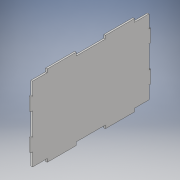
# Autodesk Inventor part: rev1 large wall
Saved by Autodesk Inventor 2017 (Build 210142000, 142)
## iProperties
Created: 2019-05-03
Part Number: rev1 large wall
Material: Generic
Document SubType Name: Modeling
Designer: Roman
Density: 1 g/cm^3
Appearance: Default
Author: Roman
Autodesk Inventor part; units mm, degrees
ref_plane "YZ Plane" through (0, 0, 0) normal (1, 0, 0) x (0, 1, 0)
sketch "Sketch1" plane through (0, 0, 0) normal (1, 0, 0) x (0, 1, 0)
  line L0 (0, 0) -> (-1168.4, 0)
  line L1 (-1168.4, 0) -> (-1168.4, -1828.8)
  line L2 (-1168.4, -1828.8) -> (0, -1828.8)
  line L3 (0, -1828.8) -> (0, 0)
  dimension "d0" = 1168.4
  dimension "d1" = 1828.8
  constraints: 8 end point, 2 parallel, 1 horizontal, 1 perpendicular
  measures "d0" distance of L2.end L1.end
  measures "d1" distance of L1.end L0.end
extrude "Extrusion1" add sketch "Sketch1" along normal blind 25.4
sketch "Sketch2" plane through (0, -1168.4, -1828.8) normal (0, -1, 0) x (1, 0, 0)
  line L0 (25.4, 1828.8) -> (25.4, 0) projected
  line L1 (0, 1828.8) -> (0, 0) projected
  line L2 (25.4, 1600.2) -> (0, 1600.2)
  line L3 (0, 1600.2) -> (0, 1143)
  line L4 (0, 1143) -> (25.4, 1143)
  line L5 (25.4, 1143) -> (25.4, 1600.2)
  line L6 (25.4, 685.8) -> (0, 685.8)
  line L7 (0, 685.8) -> (0, 228.6)
  line L8 (0, 228.6) -> (25.4, 228.6)
  line L9 (25.4, 228.6) -> (25.4, 685.8)
  line L10 (12.7, 1600.2) -> (12.7, 1143)
  line L11 (12.7, 685.8) -> (12.7, 228.6)
  line L12 (0, 1828.8) -> (25.4, 1828.8) projected
  line L13 (12.7, 1828.8) -> (12.7, 1600.2)
  line L14 (0, 0) -> (25.4, 0) projected
  line L15 (12.7, 0) -> (12.7, 228.6)
  dimension "d4" = 228.6
  dimension "d5" = 457.2
  constraints: 24 end point, 6 midpoint, 4 collinear, 4 parallel, 4 point on line, 2 horizontal, 2 perpendicular
  measures "d4" distance of L13.start L10.start
  measures "d5" distance of L10.start L10.end
extrude "Extrusion2" add sketch "Sketch2" along normal blind 50.8 contours L0 L4 L10 L2 | L10 L4 L1 L2 | L0 L8 L11 L6 | L11 L8 L1 L6
sketch "Sketch3" plane through (0, -1168.4, 0) normal (0, 0, 1) x (1, 0, 0)
  line L0 (0, 0) -> (0, 1168.4) projected
  line L1 (25.4, 0) -> (25.4, 1168.4) projected
  line L2 (0, 203.2) -> (25.4, 203.2)
  line L3 (25.4, 203.2) -> (25.4, 406.4)
  line L4 (25.4, 406.4) -> (0, 406.4)
  line L5 (0, 406.4) -> (0, 203.2)
  line L6 (0, 1168.4) -> (0, 0) projected
  line L7 (0, 0) -> (25.4, 0) projected
  line L8 (25.4, 1168.4) -> (25.4, 0) projected
  line L9 (0, 1168.4) -> (25.4, 1168.4) projected
  line L10 (0, 965.2) -> (25.4, 965.2)
  line L11 (25.4, 965.2) -> (25.4, 762)
  line L12 (25.4, 762) -> (0, 762)
  line L13 (0, 762) -> (0, 965.2)
  dimension "d8" = 203.2
  dimension "d9" = 203.2
  dimension "d12" = 203.2
  dimension "d13" = 355.6
  constraints: 16 end point, 4 parallel, 4 point on line, 2 horizontal, 2 perpendicular
  measures "d8" distance between parallel lines of L2 L7
  measures "d9" distance between parallel lines of L4 L2
  measures "d12" distance between parallel lines of L12 L10
  measures "d13" distance between parallel lines of L4 L12
extrude "Extrusion3" add sketch "Sketch3" along normal blind 25.4 contours L0 L4 L1 L2 | L0 L10 L1 L12
ref_plane "Work Plane1" through (0, 0, -914.4) normal (0, 0, 1) x (1, 0, 0)
mirror "Mirror1" about plane through (0, 0, -914.4) normal (0, 0, 1) of "Extrusion3"
ref_plane "Work Plane2" through (0, -584.2, -1143) normal (0, -1, 0) x (1, 0, 0)
mirror "Mirror2" about plane through (0, -584.2, -1143) normal (0, -1, 0) of "Extrusion2"
body "Solid1"
